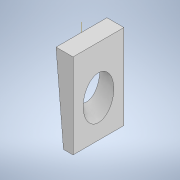
# Autodesk Inventor part: waterHeaterVent-V01
Saved by Autodesk Inventor 2021.1 (Build 251245010, 245A)
## iProperties
Created: 2020-10-25
Part Number: waterHeaterVent-V01
Material: Generic
Document SubType Name: Modeling
Designer: robst
Density: 1 g/cm^3
Appearance: Default
Author: robst
Autodesk Inventor part; units mm, degrees
ref_plane "YZ Plane" through (0, 0, 0) normal (1, 0, 0) x (0, 1, 0)
ref_plane "XZ Plane" through (0, 0, 0) normal (0, 1, 0) x (-1, 0, 0)
ref_plane "XY Plane" through (0, 0, 0) normal (0, 0, 1) x (1, 0, 0)
sketch "Sketch1" plane through (0, 0, 0) normal (0, 0, 1) x (1, 0, 0)
  line L0 (0, 0) -> (5.5555, -63.5)
  line L1 (0, -60.96) -> (0, 10.16) projected
  line L2 (0, 0) -> (12.7, 0)
  line L3 (12.7, 0) -> (12.7, -63.5)
  line L4 (5.5555, -63.5) -> (12.7, -63.5)
  dimension "d0" = 5
  dimension "d1" = 12.7
  dimension "d3" = 63.5
  constraints: 8 end point, 2 horizontal, 1 vertical
  measures "d0" angle of L0 L1
  measures "d1" distance of L0.start L2.end
  measures "d3" distance of L2.end L3.end
extrude "Extrusion1" add sketch "Sketch1" along normal mid plane 38.1
ref_plane "Work Plane1" through (12.7, -63.5, 0) normal (0.7071068, -0.7071068, 0) x (0, 0, 1)
sketch "Sketch2" plane through (12.7, -63.5, 0) normal (0.7071068, -0.7071068, 0) x (0, 0, 1)
  line L0 (19.05, 0) -> (19.05, -44.9013) projected
  line L1 (19.05, -44.9013) -> (-19.05, -44.9013) projected
  line L2 (-19.05, -44.9013) -> (-19.05, 0) projected
  line L3 (-19.05, 0) -> (19.05, 0) projected
  circle A0 centre (0, -19.5013) radius 11.43
  point P0 (0, -35.921)
  dimension "d7" = 22.86
  dimension "d10" = 25.4
  constraints: 1 centre point
  measures "d7" diameter of A0
  measures "d10" distance from line of A0.centre L1
extrude "Extrusion2" cut sketch "Sketch2" against normal through all contours A0
sketch "Sketch3" plane through (5.5555, -63.5, -19.05) normal (-0.9961947, -0.0871557, 0) x (0, 0, 1)
  line L0 (0, 0) -> (0, 63.7426) construction
  line L1 (0, 12.7) -> (38.1, 12.7) construction
  line L2 (38.1, 63.7426) -> (38.1, 0) construction
  line L3 (0, 0) -> (38.1, 0) construction
  line L4 (11.6348, 19.05) -> (7.2608, 6.35)
  line L5 (7.2608, 6.35) -> (5.4392, 6.35)
  line L6 (5.4392, 6.35) -> (1.0652, 19.05)
  line L7 (1.0652, 19.05) -> (2.8765, 19.05)
  line L8 (2.8765, 19.05) -> (6.3963, 8.501)
  line L9 (6.3963, 8.501) -> (9.9161, 19.05)
  line L10 (9.9161, 19.05) -> (11.6348, 19.05)
  line L11 (17.285, 11.1357) -> (12.4787, 11.1357)
  line L12 (12.4787, 11.1357) -> (12.4787, 12.6794)
  line L13 (12.4787, 12.6794) -> (17.285, 12.6794)
  line L14 (17.285, 12.6794) -> (17.285, 11.1357)
  spline S0 degree 2 poles (26.8769, 12.7) (26.8769, 9.2831) (24.8906, 6.0824) (22.8219, 6.0824) knots 0 0 0 1 2 2 2
  spline S1 degree 2 poles (22.8219, 6.0824) (20.7224, 6.0824) (18.7567, 9.3449) (18.7567, 12.6897) knots 0 0 0 1 2 2 2
  spline S2 degree 2 poles (18.7567, 12.6897) (18.7567, 16.1271) (20.743, 19.3073) (22.8219, 19.3073) knots 0 0 0 1 2 2 2
  spline S3 degree 2 poles (22.8219, 19.3073) (24.9111, 19.3073) (26.8769, 16.0139) (26.8769, 12.7) knots 0 0 0 1 2 2 2
  spline S4 degree 2 poles (24.695, 8.8303) (24.942, 9.4581) (25.1479, 11.3929) (25.1479, 12.7) knots 0 0 0 1 2 2 2
  spline S5 degree 2 poles (25.1479, 12.7) (25.1479, 14.0071) (24.942, 15.9316) (24.6847, 16.58) knots 0 0 0 1 2 2 2
  spline S6 degree 2 poles (24.6847, 16.58) (24.4274, 17.2284) (23.5321, 17.8973) (22.8219, 17.8973) knots 0 0 0 1 2 2 2
  spline S7 degree 2 poles (22.8219, 17.8973) (22.1118, 17.8973) (21.1958, 17.2284) (20.9282, 16.5594) knots 0 0 0 1 2 2 2
  spline S8 degree 2 poles (20.9282, 16.5594) (20.6709, 15.911) (20.4857, 13.935) (20.4857, 12.6897) knots 0 0 0 1 2 2 2
  spline S9 degree 2 poles (20.4857, 12.6897) (20.4857, 11.3518) (20.6504, 9.561) (20.918, 8.8612) knots 0 0 0 1 2 2 2
  spline S10 degree 2 poles (20.918, 8.8612) (21.165, 8.2025) (22.0809, 7.4924) (22.8219, 7.4924) knots 0 0 0 1 2 2 2
  spline S11 degree 2 poles (22.8219, 7.4924) (23.5218, 7.4924) (24.4377, 8.1613) (24.695, 8.8303) knots 0 0 0 1 2 2 2
  line L15 (35.6969, 6.35) -> (29.5013, 6.35)
  line L16 (29.5013, 6.35) -> (29.5013, 7.6468)
  line L17 (29.5013, 7.6468) -> (31.8066, 7.6468)
  line L18 (31.8066, 7.6468) -> (31.8066, 16.158)
  line L19 (31.8066, 16.158) -> (29.5013, 16.158)
  line L20 (29.5013, 16.158) -> (29.5013, 17.321)
  spline S12 degree 2 poles (29.5013, 17.321) (30.8083, 17.321) (32.0433, 18.062) (32.1256, 19.0912) knots 0 0 0 1 2 2 2
  line L21 (32.1256, 19.0912) -> (33.443, 19.0912)
  line L22 (33.443, 19.0912) -> (33.443, 7.6468)
  line L23 (33.443, 7.6468) -> (35.6969, 7.6468)
  line L24 (35.6969, 7.6468) -> (35.6969, 6.35)
  point P0 (19.05, 63.7426)
  dimension "d12" = 12.7
  constraints: 2 end point, 2 horizontal, 2 point on line
  measures "d12" distance between parallel lines of L3 L1
extrude "Extrusion3" cut sketch "Sketch3" against normal blind 1.27
equation "\"d0\" = backAngle"
equation "\"d1\" = topPartDepth"
equation "\"d3\" = partHeight"
equation "\"d4\" = partWidth"
equation "\"d7\" = pipeExteriorDiameter"
equation "\"d10\" = pipeCenter"
equation "\"topPartDepth\" = 12.7"
equation "\"backAngle\" = 5deg"
equation "\"partHeight\" = 63.5"
equation "\"partWidth\" = 38.1"
equation "\"pipeExteriorDiameter\" = 22.86"
equation "\"pipeCenter\" = 25.4"
equation "\"filletEdge\" = 1.05833"
body "Solid1"
